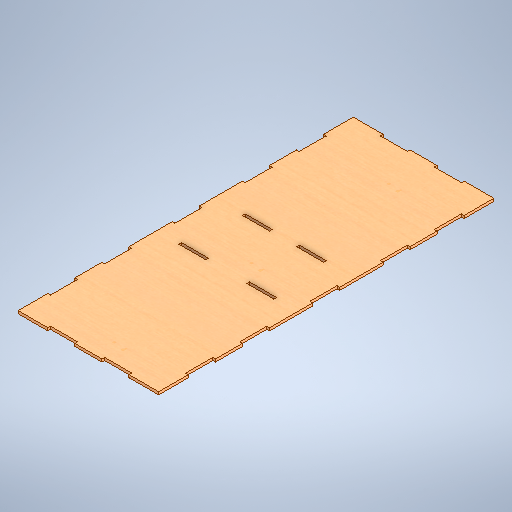
# Autodesk Inventor part: Base
Saved by Autodesk Inventor 2025 (Build 290162000, 162)
## iProperties
Created: 2024-11-02
Part Number: Base
Material: Wood (Cherry)
Document SubType Name: Sheet Metal
Designer: g.marin
Density: 0.63 g/cm^3
Sheet Metal Rule: Default
Appearance: Cherry - Natural Low Gloss
Author: g.marin
Autodesk Inventor part; units mm, degrees
ref_plane "YZ Plane" through (0, 0, 0) normal (1, 0, 0) x (0, 1, 0)
ref_plane "XZ Plane" through (0, 0, 0) normal (0, 1, 0) x (-1, 0, 0)
ref_plane "XY Plane" through (0, 0, 0) normal (0, 0, 1) x (1, 0, 0)
sketch "Sketch1" plane through (0, 0, 0) normal (0, 1, 0) x (-1, 0, 0)
  line L0 (260, 360) -> (0, 360)
  line L1 (0, 360) -> (0, 100)
  line L2 (0, 100) -> (260, 100)
  line L3 (260, 100) -> (260, 360)
  line L4 (260, 0) -> (0, 0)
  line L5 (0, 0) -> (0, -260)
  line L6 (0, -260) -> (260, -260)
  line L7 (260, -260) -> (260, 0)
  line L8 (260, 100) -> (0, 100)
  line L9 (0, 100) -> (0, 0)
  line L10 (0, 0) -> (260, 0)
  line L11 (260, 0) -> (260, 100)
  line L12 (260, 25) -> (255, 25)
  line L13 (255, 25) -> (255, 75)
  line L14 (255, 75) -> (260, 75)
  line L15 (260, 75) -> (260, 25)
  line L16 (260, 155) -> (255, 155)
  line L17 (255, 155) -> (255, 205)
  line L18 (255, 205) -> (260, 205)
  line L19 (260, 205) -> (260, 155)
  line L20 (260, 255) -> (255, 255)
  line L21 (255, 255) -> (255, 305)
  line L22 (255, 305) -> (260, 305)
  line L23 (260, 305) -> (260, 255)
  line L24 (130, -260) -> (130, 360) construction
  line L25 (260, 50) -> (0, 50) construction
  line L26 (260, -55) -> (255, -55)
  line L27 (255, -55) -> (255, -105)
  line L28 (255, -105) -> (260, -105)
  line L29 (260, -155) -> (255, -155)
  line L30 (255, -155) -> (255, -205)
  line L31 (255, -205) -> (260, -205)
  line L32 (0, 25) -> (5, 25)
  line L33 (5, 25) -> (5, 75)
  line L34 (5, 75) -> (0, 75)
  line L35 (0, 155) -> (5, 155)
  line L36 (5, 155) -> (5, 205)
  line L37 (5, 205) -> (0, 205)
  line L38 (0, 255) -> (5, 255)
  line L39 (5, 255) -> (5, 305)
  line L40 (5, 305) -> (0, 305)
  line L41 (5, -55) -> (5, -105)
  line L42 (5, -105) -> (0, -105)
  line L43 (0, -55) -> (5, -55)
  line L44 (5, -205) -> (0, -205)
  line L45 (5, -155) -> (5, -205)
  line L46 (0, -155) -> (5, -155)
  line L47 (205, -260) -> (155, -260)
  line L48 (155, -260) -> (155, -255)
  line L49 (155, -255) -> (205, -255)
  line L50 (205, -255) -> (205, -260)
  line L51 (105, -260) -> (55, -260)
  line L52 (55, -260) -> (55, -255)
  line L53 (55, -255) -> (105, -255)
  line L54 (105, -255) -> (105, -260)
  line L55 (155, 360) -> (155, 355)
  line L56 (155, 355) -> (205, 355)
  line L57 (205, 355) -> (205, 360)
  line L58 (55, 360) -> (55, 355)
  line L59 (55, 355) -> (105, 355)
  line L60 (105, 355) -> (105, 360)
  line L61 (260, -130) -> (0, -130) construction
  line L62 (260, 230) -> (0, 230) construction
  line L63 (155, 0) -> (155, -5)
  line L64 (155, -5) -> (205, -5)
  line L65 (205, -5) -> (205, 0)
  line L66 (55, 0) -> (55, -5)
  line L67 (55, -5) -> (105, -5)
  line L68 (105, -5) -> (105, 0)
  line L69 (218, 100) -> (168, 100)
  line L70 (168, 100) -> (168, 105)
  line L71 (168, 105) -> (218, 105)
  line L72 (218, 105) -> (218, 100)
  line L73 (92, 100) -> (42, 100)
  line L74 (42, 100) -> (42, 105)
  line L75 (42, 105) -> (92, 105)
  line L76 (92, 105) -> (92, 100)
  point P0 (257.5, 255)
  point P1 (92, 102.5)
  point P2 (168, 102.5)
  point P3 (130, 100)
  dimension "d0" = 260
  dimension "d1" = 260
  dimension "d2" = 260
  dimension "d3" = 100
  dimension "d6" = 50
  dimension "d7" = 50
  dimension "d8" = 50
  dimension "d9" = 50
  dimension "d10" = 55
  dimension "d12" = 5
  dimension "d13" = 25
  dimension "d14" = 5
  dimension "d15" = 55
  dimension "d16" = 50
  dimension "d17" = 50
  dimension "d18" = 50
  dimension "d19" = 50
  dimension "d20" = 50
  dimension "d21" = 5
  dimension "d22" = 76
  dimension "d23" = 38
  constraints: 154 end point, 44 symmetric about line, 20 parallel, 19 point on line, 12 midpoint, 11 perpendicular, 10 horizontal, 1 coincident
  measures "d0" distance of L2.end L0.start
  measures "d1" distance of L0.start L0.end
  measures "d2" distance of L6.end L4.start
  measures "d3" distance of L10.end L2.end
  measures "d6" distance of L12.end L13.end
  measures "d7" distance of L16.end L17.end
  measures "d8" distance of L20.end L21.end
  measures "d9" distance from line of point (257.5, 255) L18
  measures "d10" distance between parallel lines of L0 L22
  measures "d12" distance between parallel lines of L13 L15
  measures "d13" distance between parallel lines of L12 L4
  measures "d14" distance between parallel lines of L49 L6
  measures "d15" distance between parallel lines of L50 L7
  measures "d16" distance of L48.end L49.end
  measures "d17" distance of L52.end L53.end
  measures "d18" distance between parallel lines of L54 L48
  measures "d19" distance of L70.end L71.end
  measures "d20" distance of L74.end L75.end
  measures "d21" distance of L69.end L70.end
  measures "d22" distance of point (92, 102.5) point (168, 102.5)
  measures "d23" horizontal distance of point (130, 100) L70.end
extrude "Extrusion1" add sketch "Sketch1" along normal blind 5 contours L3 L22 L21 L20 L18 L17 L16 L2 L72 L71 L70 L76 L75 L74 L1 L35 L36 L37 L38 L39 L40 L0 L58 L59 L60 L55 L56 L57 | L11 L14 L13 L12 L4 L9 L32 L33 L34 L2 | L7 L26 L27 L28 L29 L30 L31 L6 L50 L49 L48 L54 L53 L52 L5 L44 L45 L46 L42 L41 L43 L4 L66 L67 L68 L63 L64 L65
equation "\"BendRadius\" = Thickness"
equation "\"BendReliefWidth\" = Thickness"
equation "\"BendReliefDepth\" = 0.5 * Thickness"
equation "\"CornerReliefSize\" = 4 * Thickness"
equation "\"MinimumRemnant\" = 2 * Thickness"
equation "\"TransitionRadius\" = BendRadius"
equation "\"JacobiRadiusSize\" = BendRadius"
equation "\"GapSize\" = Thickness"
equation "\"Thickness\" = 3.048"
body "Solid1"
